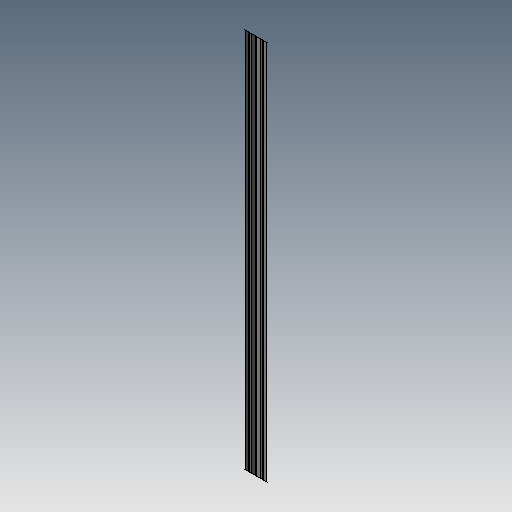
# Autodesk Inventor part: HFS6-3030-1005.5-LAT45-RCT45
Saved by Autodesk Inventor 2020 (Build 240168000, 168)
## iProperties
Part Number: HFS6-3030-1005.5-LAT45-RCT45
Material: 一般
Catalog Web Link: www.cadenas.de
Description: NEFS6-3030, NEFSB6-3030, EFS6-3030, EFSB6-3030, HFS6-3030, HFSB6-3030, CAF6-3030, HFSY6-3030, NFSL6-3030,  HFSL6-3030, HFSLB6-3030, GFS6-3030-HFS6 Series Aluminum Extrusions 30 Square -1 Slot-
Vendor: MISUMI
Document SubType Name: Modeling
Designer: partserver
Manufacturer: MISUMI
Mass: 323.782 g
Surface Area: 3074.21 cm^2
Volume: 323.782 cm^3
Density: 1 g/cm^3
Appearance: PSOLRGB-175-175-175
Category: PARTsolutions
Company: MISUMI
PSOL_IDENT_0: {$CADENAS_DATA\23d-libs\misumi\metric\38_al_extrusions_blackets\6\hfs6_3030.prj},750 {VTYP=3D},{NB=H
PSOL_IDENT_1: FS6-3030-1005.5-LAT45-RCT45},{LINA=HFS6-3030-1005.5-LAT45-RCT45},{NN=NEFS6-3030, NEFSB6-3030, EFS6-3
PSOL_IDENT_2: 030, EFSB6-3030, HFS6-3030, HFSB6-3030, CAF6-3030, HFSY6-3030, NFSL6-3030,  HFSL6-3030, HFSLB6-3030,
PSOL_IDENT_3: GFS6-3030},{DATE=30.06.2021 13:36:38},{GEOMDATE=08.06.2016 01:16:00},{VERSION=},{LINEID=130},{WBVAR=
PSOL_IDENT_4: L,ALT1,ALT2,ALT3,ALT4,ALT5,CP5,DL5,DR5,ALT6,ALT9,ALT10,ALT11,DD6SE,DD6,HP6,NHL6,DL6,NHR6,DR6,ALT7,AL
PSOL_IDENT_5: T8,NH9,AH,BH,CH,DH,EH,NH10,AV,BV,CV,DV,EV,NH11,AP,BP,CP,DP,EP,ALT12,ALT13,Z,NH12,XA,XB,XC,XD,XE,NH13
PSOL_IDENT_6: ,YA,YB,YC,YD,YE,ALT14,HP14,DL14,DR14,ALT15,HP15,DL15,DR15,ALT16,HP16,DL16,DR16,ALT17,HQ17,JLP,ALT19,
PSOL_IDENT_7: ALT20},{WBNUMERIC=L,DD6,NH9,AH,BH,CH,DH,EH,NH10,AV,BV,CV,DV,EV,NH11,AP,BP,CP,DP,EP,NH12,XA,XB,XC,XD,
PSOL_IDENT_8: XE,NH13,YA,YB,YC,YD,YE,HQ17,JLP}  {NB=HFS6-3030-1005.5-LAT45-RCT45},{LINA=HFS6-3030-1005.5-LAT45-RCT
PSOL_IDENT_9: 45},{KT=DUMMY},{PN=HFS6-3030-1005.5-LAT45-RCT45},{TPS=HFS6-3030},{MAT=A6N01SS-T5 Aluminum Alloy},{ST=
PSOL_IDENT_10: Clear Anodize},{FRMW=30},{FRMH=30},{FRD=6.8},{L=1005.5},{MASS=0.90},{SA=333},{LX=2.83x10^4},{LY=2.83
PSOL_IDENT_11: x10^4},{ALT1=},{M1=0},{IDM1=6.647},{DALT1=4.2},{DPL1=0},{DPR1=0},{ALT1PN=},{ALT2=},{ALT2ALG= '','w/o
PSOL_IDENT_12: End Tapping (Heli-Coil Insert)','LHP','with LHP (Tapping on the Left (Heli-Coil Insert))','RHP','wi
PSOL_IDENT_13: th RHP (Tapping on the Right (Heli-Coil Insert))','HPW','with HPW (Tapping on Both Ends (Heli-Coil I
PSOL_IDENT_14: nsert))' },{M2=0},{DP2=0},{ALT2PN=},{ALT3=},{ALT3ALG= '','w/o Tapping (Corner Section)','LSP','with
PSOL_IDENT_15: LSP (Tapping (Corner Section))','RSP','with RSP (Tapping (Corner Section))','SPW','with SPW (Tapping
PSOL_IDENT_16: (Corner Section))' },{M3=0},{IDM3=4.134},{DP3=0},{ALT3PN=},{ALT4=},{ALT4ALG= '', 'w/o SC (High Prec
PSOL_IDENT_17: ision Cut)', 'SC', 'with SC (High Precision Cut)' },{ALT4PN=},{ALT5=1},{ALT5ALG= '','w/o 45 Degree C
PSOL_IDENT_18: ut','1','with 45 Degree Cut' },{CP5=LR},{CP5ALG= 'L','Left End','R','Right End','LR','Both Ends' },{
PSOL_IDENT_19: DL5=A},{DL5ALG= 'A','A (Cut with cross the section facing down)','B','B (Cut with cross the section
PSOL_IDENT_20: facing back)','C','C (Cut with cross the section facing up)','D','D (Cut with cross the section faci
PSOL_IDENT_21: ng front)' },{DR5=C},{DR5ALG= 'A','A (Cut with cross the section facing down)','B','B (Cut with cros
PSOL_IDENT_22: s the section facing back)','C','C (Cut with cross the section facing up)','D','D (Cut with cross th
PSOL_IDENT_23: e section facing front)' },{FRMLALT5=30},{FRMRALT5=30},{ALT5PN=-LAT45-RCT45},{ALT6=},{ALT6ALG= '','w
PSOL_IDENT_24: /o Fastening Location Wrench Access Hole Alterations','1','with Fastening Location Wrench Access Hol
PSOL_IDENT_25: e Alterations' },{ALT9=},{ALT9ALG= '','w/o Location Specified Wrench Access Hole Alteratons (Horizon
PSOL_IDENT_26: tal)','1','with Location Specified Wrench Access Hole Alteratons (Horizontal)' },{ALT10=},{ALT10ALG=
PSOL_IDENT_27: '','w/o Location Specified Wrench Access Hole Alteratons (Vertical)','1','with Location Specified W
PSOL_IDENT_28: rench Access Hole Alteratons (Vertical)' },{ALT11=},{ALT11ALG= '','w/o Location Specified Wrench Acc
PSOL_IDENT_29: ess Hole Alteratons (Crisscross)','1','with Location Specified Wrench Access Hole Alteratons (Crissc
PSOL_IDENT_30: ross)' },{DD6SE=},{DD6SEALG= '','N/A' },{DD6=0},{DD6ALG=0},{HP6=},{HP6ALG= '','N/A' },{NHL6=},{NHL6A
PSOL_IDENT_31: LG= '','N/A' },{DL6=},{DL6ALG= '','N/A' },{NHR6=},{NHR6ALG= '','N/A' },{DR6=},{DR6ALG= '','N/A' },{D
PSOL_IDENT_32: D6PN=},{HL6=0},{HL6D=0},{HR6=0},{HR6D=0},{J6=0},{J6D=0},{K6=0},{K6D=0},{ALT7=},{ALT7ALG= '','N/A' },
PSOL_IDENT_33: {ALT8=},{ALT8ALG= '','N/A' },{ALT678PN=},{NH9=0},{NH9MAX=5},{NH9ALG=[0]},{AH=0.0},{AHMIN=7},{AHMAX=1
PSOL_IDENT_34: 000.5},{AHALG=[0]},{BH=0.0},{BHMIN=2},{BHMAX=1002.5},{BHALG=[0]},{CH=0.0},{CHMIN=2},{CHMAX=1004.5},{
PSOL_IDENT_35: CHALG=[0]},{DH=0.0},{DHMIN=2},{DHMAX=1006.5},{DHALG=[0]},{EH=0.0},{EHMIN=2},{EHMAX=998.5},{EHALG=[0]
PSOL_IDENT_36: },{NH10=0},{NH10MAX=5},{NH10ALG=[0]},{AV=0.0},{AVMIN=7},{AVMAX=1000.5},{AVALG=[0]},{BV=0.0},{BVMIN=2
PSOL_IDENT_37: },{BVMAX=1002.5},{BVALG=[0]},{CV=0.0},{CVMIN=2},{CVMAX=1004.5},{CVALG=[0]},{DV=0.0},{DVMIN=2},{DVMAX=
PSOL_IDENT_38: 1006.5},{DVALG=[0]},{EV=0.0},{EVMIN=2},{EVMAX=998.5},{EVALG=[0]},{NH11=0},{NH11MAX=5},{NH11ALG=[0]},
PSOL_IDENT_39: {AP=0.0},{APMIN=7},{APMAX=1000.5},{APALG=[0]},{BP=0.0},{BPMIN=2},{BPMAX=1002.5},{BPALG=[0]},{CP=0.0}
PSOL_IDENT_40: ,{CPMIN=2},{CPMAX=1004.5},{CPALG=[0]},{DP=0.0},{DPMIN=2},{DPMAX=1006.5},{DPALG=[0]},{EP=0.0},{EPMIN=
PSOL_IDENT_41: 2},{EPMAX=998.5},{EPALG=[0]},{ALT9PN=},{ALT10PN=},{ALT11PN=},{ALT91011PN=},{ALT12=},{ALT12ALG= '','w
PSOL_IDENT_42: /o Counterbore Hole in Specified Position (Vertical)','1','with Counterbore Hole in Specified Positi
PSOL_IDENT_43: on (Vertical)' },{ALT13=},{ALT13ALG= '','w/o Counterbore Hole in Specified Position (Horizontal)','1'
PSOL_IDENT_44: ,'with Counterbore Hole in Specified Position (Horizontal)' },{Z=},{ZALG= '','N/A' },{DD12=0.0},{DD1
PSOL_IDENT_45: 12=0.0},{NH12=0},{NH12MAX=5},{NH12ALG=[0]},{XA=0.0},{XAMIN=7},{XAMAX=1000.5},{XAALG=[0]},{XB=0.0},{X
PSOL_IDENT_46: BMIN=2},{XBMAX=1002.5},{XBALG=[0]},{XC=0.0},{XCMIN=2},{XCMAX=1004.5},{XCALG=[0]},{XD=0.0},{XDMIN=2},
PSOL_IDENT_47: {XDMAX=1006.5},{XDALG=[0]},{XE=0.0},{XEMIN=2},{XEMAX=998.5},{XEALG=[0]},{NH13=0},{NH13MAX=5},{NH13AL
PSOL_IDENT_48: G=[0]},{YA=0.0},{YAMIN=7},{YAMAX=1000.5},{YAALG=[0]},{YB=0.0},{YBMIN=2},{YBMAX=1002.5},{YBALG=[0]},{
PSOL_IDENT_49: YC=0.0},{YCMIN=2},{YCMAX=1004.5},{YCALG=[0]},{YD=0.0},{YDMIN=2},{YDMAX=1006.5},{YDALG=[0]},{YE=0.0},
PSOL_IDENT_50: {YEMIN=2},{YEMAX=998.5},{YEALG=[0]},{ALT12PN=},{ALT13PN=},{ALT1213PN=},{ALT14=},{ALT14ALG= '','w/o D
PSOL_IDENT_51: Type Hole Alteration','1','with D Type Hole Alteration' },{HP14=},{HP14ALG= '','N/A' },{DL14=},{DL1
PSOL_IDENT_52: 4ALG= '','N/A' },{DR14=},{DR14ALG= '','N/A' },{H14=0},{D14=0.0},{ALT14PN=},{ALT15=},{ALT15ALG= '','w
PSOL_IDENT_53: /o S Type Hole Alteration','1','with S Type Hole Alteration' },{HP15=},{HP15ALG= '','N/A' },{DL15=},
PSOL_IDENT_54: {DL15ALG= '','N/A' },{DR15=},{DR15ALG= '','N/A' },{H15=0},{D115=0.0},{D215=0.0},{ALT15PN=},{ALT16=},
PSOL_IDENT_55: {ALT16ALG= '','w/o M Type Hole Alteration','1','with M Type Hole Alteration' },{HP16=},{HP16ALG= '','
PSOL_IDENT_56: N/A' },{DL16=},{DL16ALG= '','N/A' },{DR16=},{DR16ALG= '','N/A' },{H116=0},{D16=0.0},{ALT16PN=},{ALT1
PSOL_IDENT_57: 7=},{ALT17ALG= '','w/o L Type Hole Alteration (Top)','1','with L Type Hole Alteration (Top)' },{HQ17=
PSOL_IDENT_58: 0},{HQ17ALG=0},{JLP=0},{JLPMIN=4.9},{JLPMAX=0},{JLPALG=[0]},{L17=0},{D17=0.0},{ALT17PN=},{ALT19=},{A
PSOL_IDENT_59: LT19ALG= '','N/A' },{M19=0},{DP19=0},{ALT19PN=},{ALT20=},{ALT20PN=},{ERRORALT01=OK},{ERRORALT02=OK},
PSOL_IDENT_60: {ERRORALT03=OK},{ERRORALT05=OK},{ERRORALT06091=OK},{ERRORALT06092=OK},{ERRORALT06093=OK},{ERRORALT06
PSOL_IDENT_61: 094=OK},{ERRORALT06101=OK},{ERRORALT06102=OK},{ERRORALT06103=OK},{ERRORALT06104=OK},{ERRORALT06111=O
PSOL_IDENT_62: K},{ERRORALT06112=OK},{ERRORALT06113=OK},{ERRORALT06114=OK},{ERRORALT06121=OK},{ERRORALT06122=OK},{E
PSOL_IDENT_63: RRORALT06123=OK},{ERRORALT06124=OK},{ERRORALT06131=OK},{ERRORALT06132=OK},{ERRORALT06133=OK},{ERRORA
PSOL_IDENT_64: LT06134=OK},{ERRORALT0614=OK},{ERRORALT0615=OK},{ERRORALT0616=OK},{ERRORALT06171=OK},{ERRORALT06172=
PSOL_IDENT_65: OK},{ERRORALT06173=OK},{ERRORALT0619=OK},{ERRORALT0911=OK},{ERRORALT0913=OK},{ERRORALT0914=OK},{ERRO
PSOL_IDENT_66: RALT0915=OK},{ERRORALT0916=OK},{ERRORALT0917=OK},{ERRORALT0919=OK},{ERRORALT1011=OK},{ERRORALT1012=O
PSOL_IDENT_67: K},{ERRORALT1014=OK},{ERRORALT1015=OK},{ERRORALT1016=OK},{ERRORALT1017=OK},{ERRORALT1019=OK},{ERRORA
PSOL_IDENT_68: LT1112=OK},{ERRORALT1113=OK},{ERRORALT1114=OK},{ERRORALT1115=OK},{ERRORALT1116=OK},{ERRORALT1117=OK}
PSOL_IDENT_69: ,{ERRORALT1119=OK},{ERRORALT1214=OK},{ERRORALT1215=OK},{ERRORALT1216=OK},{ERRORALT1217=OK},{ERRORALT
PSOL_IDENT_70: 1219=OK},{ERRORALT1314=OK},{ERRORALT1315=OK},{ERRORALT1316=OK},{ERRORALT1317=OK},{ERRORALT1319=OK},{
PSOL_IDENT_71: ERRORALT1415=OK},{ERRORALT1416=OK},{ERRORALT1417=OK},{ERRORALT1419=OK},{ERRORALT1516=OK},{ERRORALT15
PSOL_IDENT_72: 17=OK},{ERRORALT1519=OK},{ERRORALT1617=OK},{ERRORALT1619=OK},{ERRORALT1719=OK},{ERRORPN=}
NB: HFS6-3030-1005.5-LAT45-RCT45
NN: NEFS6-3030, NEFSB6-3030, EFS6-3030, EFSB6-3030, HFS6-3030, HFSB6-3030, CAF6-3030, HFSY6-3030, NFSL6-3030,  HFSL6-3030, HFSLB6-3030, GFS6-3030
NT: HFS6 Series Aluminum Extrusions 30 Square -1 Slot-
NBSYN: $PN.
LINA: HFS6-3030-1005.5-LAT45-RCT45
CATALOG: Misumi
PN: HFS6-3030-1005.5-LAT45-RCT45
TPS: HFS6-3030
MAT: A6N01SS-T5 Aluminum Alloy
ST: Clear Anodize
L: 1005.5
MASS: 0.90
SA: 333
LX: 2.83x10^4
LY: 2.83x10^4
ALT1: w/o End Tapping
M1: 0
DPL1: 0
DPR1: 0
ALT2: w/o End Tapping (Heli-Coil Insert)
M2: 0
DP2: 0
ALT3: w/o Tapping (Corner Section)
M3: 0
DP3: 0
ALT4: w/o SC (High Precision Cut)
ALT5: with 45 Degree Cut
CP5: Both Ends
DL5: A (Cut with cross the section facing down)
DR5: C (Cut with cross the section facing up)
ALT6: w/o Fastening Location Wrench Access Hole Alterations
ALT9: w/o Location Specified Wrench Access Hole Alteratons (Horizontal)
ALT10: w/o Location Specified Wrench Access Hole Alteratons (Vertical)
ALT11: w/o Location Specified Wrench Access Hole Alteratons (Crisscross)
DD6SE: N/A
DD6: 0
HP6: N/A
NHL6: N/A
DL6: N/A
NHR6: N/A
DR6: N/A
HL6D: 0
HR6D: 0
J6D: 0
K6D: 0
ALT7: N/A
ALT8: N/A
NH9: 0
AH: 0
BH: 0
CH: 0
DH: 0
EH: 0
NH10: 0
AV: 0
BV: 0
CV: 0
DV: 0
EV: 0
NH11: 0
AP: 0
BP: 0
CP: 0
DP: 0
EP: 0
ALT12: w/o Counterbore Hole in Specified Position (Vertical)
ALT13: w/o Counterbore Hole in Specified Position (Horizontal)
Z: N/A
DD12: 0
DD112: 0
NH12: 0
XA: 0
XB: 0
XC: 0
XD: 0
XE: 0
NH13: 0
YA: 0
YB: 0
YC: 0
YD: 0
YE: 0
ALT14: w/o D Type Hole Alteration
HP14: N/A
DL14: N/A
DR14: N/A
H14: 0
D14: 0
ALT15: w/o S Type Hole Alteration
HP15: N/A
DL15: N/A
DR15: N/A
H15: 0
D115: 0
D215: 0
ALT16: w/o M Type Hole Alteration
HP16: N/A
DL16: N/A
DR16: N/A
H116: 0
D16: 0
ALT17: w/o L Type Hole Alteration (Top)
HQ17: 0
JLP: 0
D17: 0
ALT19: N/A
M19: 0
DP19: 0
ALT20: w/o CW (End Face C Chamfering)
SUPPLIER: MISUMI
ARTICLENO: HFS6-3030-1005.5-LAT45-RCT45
BOMINFO: HFS6-3030-1005.5-LAT45-RCT45
CREATOR: CADENAS GmbH
Title: HFS6-3030-1005.5-LAT45-RCT45
Author: Cadenas PARTsolutions
Comments: HFS6 Series Aluminum Extrusions 30 Square -1 Slot-
Autodesk Inventor part; units mm, degrees
sketch "Sketch_1" plane through (0, 0, 0) normal (0, 0, 1) x (1, 0, 0)
  line L0 (-15, -4) -> (-15, -13)
  arc A0 (-15, -13) -> (-13, -15) centre (-13, -13) ccw
  line L1 (-13, -15) -> (-4, -15)
  line L2 (-4, -15) -> (-4, -13)
  line L3 (-4, -13) -> (-8.25, -13)
  line L4 (-8.25, -13) -> (-8.25, -9.6642)
  line L5 (-8.25, -9.6642) -> (-4.5858, -6)
  line L6 (-4.5858, -6) -> (-0.5196, -6)
  line L7 (-0.5196, -6) -> (0, -5.7)
  line L8 (0, -5.7) -> (0.5196, -6)
  line L9 (0.5196, -6) -> (4.5858, -6)
  line L10 (4.5858, -6) -> (8.25, -9.6642)
  line L11 (8.25, -9.6642) -> (8.25, -13)
  line L12 (8.25, -13) -> (4, -13)
  line L13 (4, -13) -> (4, -15)
  line L14 (4, -15) -> (13, -15)
  arc A1 (13, -15) -> (15, -13) centre (13, -13) ccw
  line L15 (15, -13) -> (15, -4)
  line L16 (15, -4) -> (13, -4)
  line L17 (13, -4) -> (13, -8.25)
  line L18 (13, -8.25) -> (9.6642, -8.25)
  line L19 (9.6642, -8.25) -> (6, -4.5858)
  line L20 (6, -4.5858) -> (6, -0.5196)
  line L21 (6, -0.5196) -> (5.7, 0)
  line L22 (5.7, 0) -> (6, 0.5196)
  line L23 (6, 0.5196) -> (6, 4.5858)
  line L24 (6, 4.5858) -> (9.6642, 8.25)
  line L25 (9.6642, 8.25) -> (13, 8.25)
  line L26 (13, 8.25) -> (13, 4)
  line L27 (13, 4) -> (15, 4)
  line L28 (15, 4) -> (15, 13)
  arc A2 (15, 13) -> (13, 15) centre (13, 13) ccw
  line L29 (13, 15) -> (4, 15)
  line L30 (4, 15) -> (4, 13)
  line L31 (4, 13) -> (8.25, 13)
  line L32 (8.25, 13) -> (8.25, 9.6642)
  line L33 (8.25, 9.6642) -> (4.5858, 6)
  line L34 (4.5858, 6) -> (0.5196, 6)
  line L35 (0.5196, 6) -> (0, 5.7)
  line L36 (0, 5.7) -> (-0.5196, 6)
  line L37 (-0.5196, 6) -> (-4.5858, 6)
  line L38 (-4.5858, 6) -> (-8.25, 9.6642)
  line L39 (-8.25, 9.6642) -> (-8.25, 13)
  line L40 (-8.25, 13) -> (-4, 13)
  line L41 (-4, 13) -> (-4, 15)
  line L42 (-4, 15) -> (-13, 15)
  arc A3 (-13, 15) -> (-15, 13) centre (-13, 13) ccw
  line L43 (-15, 13) -> (-15, 4)
  line L44 (-15, 4) -> (-13, 4)
  line L45 (-13, 4) -> (-13, 8.25)
  line L46 (-13, 8.25) -> (-9.6642, 8.25)
  line L47 (-9.6642, 8.25) -> (-6, 4.5858)
  line L48 (-6, 4.5858) -> (-6, 0.5196)
  line L49 (-6, 0.5196) -> (-5.7, 0)
  line L50 (-5.7, 0) -> (-6, -0.5196)
  line L51 (-6, -0.5196) -> (-6, -4.5858)
  line L52 (-6, -4.5858) -> (-9.6642, -8.25)
  line L53 (-9.6642, -8.25) -> (-13, -8.25)
  line L54 (-13, -8.25) -> (-13, -4)
  line L55 (-13, -4) -> (-15, -4)
  constraints: 112 end point, 8 point on circle, 4 centre point
extrude "Extrusion1" add sketch "Sketch_1" against normal blind 1005.5
sketch "Sketch2" plane through (0, 0, -1005.5) normal (0, 0, -1) x (-1, 0, 0)
  point P0 (0, 0)
hole "Hole1" at (0, 0, -1005.5) direction (0, 0, 1) diameter 6.8 depth 1005.5
sketch "Sketch3" plane through (0, 0, -1005.5) normal (0, 0, -1) x (-1, 0, 0)
  point P0 (-11.6, 11.6)
hole "Hole2" at (11.6, 11.6, -1005.5) direction (0, 0, 1) diameter 4.2 depth 1005.5
pattern_linear "Rectangular Pattern1" count 2 spacing 23.2 along (-1, 0, 0) count 2 spacing 23.2 along (0, -1, 0) of "Hole2"
sketch "Sketch_5" plane through (0, 0, 0) normal (1, 0, 0) x (0, 0, -1)
  line L0 (0, 15) -> (0, -15)
  line L1 (0, -15) -> (30, -15)
  line L2 (30, -15) -> (0, 15)
  constraints: 6 end point
extrude "Extrusion2" cut sketch "Sketch_5" along normal mid plane 30
sketch "Sketch_8" plane through (0, 0, 0) normal (1, 0, 0) x (0, 0, -1)
  line L0 (975.5, 15) -> (1005.5, -15)
  line L1 (1005.5, -15) -> (1005.5, 15)
  line L2 (1005.5, 15) -> (975.5, 15)
  constraints: 6 end point
extrude "Extrusion3" cut sketch "Sketch_8" along normal mid plane 30
ref_plane "C1_XY" through (0, 0, 0) normal (0, 0, 1) x (1, 0, 0)
ref_plane "C1_YZ" through (0, 0, 0) normal (1, 0, 0) x (0, 1, 0)
ref_plane "C1_ZX" through (0, 0, 0) normal (0, 1, 0) x (0, 0, 1)
ref_plane "to_frame_cap1_XY" through (0, 0, 0) normal (0, 0, 1) x (1, 0, 0)
ref_plane "to_frame_cap1_YZ" through (0, 0, 0) normal (1, 0, 0) x (0, 1, 0)
ref_plane "to_frame_cap1_ZX" through (0, 0, 0) normal (0, 1, 0) x (0, 0, 1)
ref_plane "to_frame_cap2_XY" through (0, 0, -1005.5) normal (0, 0, -1) x (1, 0, 0)
ref_plane "to_frame_cap2_YZ" through (0, 0, -1005.5) normal (1, 0, 0) x (0, -1, 0)
ref_plane "to_frame_cap2_ZX" through (0, 0, -1005.5) normal (0, -1, 0) x (0, 0, -1)
body "Solid1"
